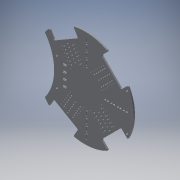
# Autodesk Inventor part: Bottom Plate
Saved by Autodesk Inventor 2016 (Build 200138000, 138)
## iProperties
Created: 2015-08-20
Part Number: Bottom Plate
Material: Generic
Document SubType Name: Modeling
Designer: TFHulbert
Density: 1 g/cm^3
Appearance: Default
Author: TFHulbert
Autodesk Inventor part; units mm, degrees
ref_plane "YZ Plane" through (0, 0, 0) normal (1, 0, 0) x (0, 1, 0)
ref_plane "XZ Plane" through (0, 0, 0) normal (0, 1, 0) x (-1, 0, 0)
ref_plane "XY Plane" through (0, 0, 0) normal (0, 0, 1) x (1, 0, 0)
sketch "Sketch1" plane through (0, 0, 0) normal (0, 1, 0) x (-1, 0, 0)
  arc A0 (31.5311, 101.5419) -> (30.2114, 104.4989) centre (29.799, 102.5419) ccw
  arc A1 (-38.945, 95.3943) -> (-39.4544, 92.1964) centre (-38.0402, 93.6107) ccw
  arc A2 (-81.8808, 49.77) -> (-85.0786, 49.2607) centre (-83.295, 48.3558) ccw
  arc A3 (30.2114, -100.9882) -> (31.5311, -98.0311) centre (29.799, -99.0311) ccw
  arc A4 (86.7133, -68.3668) -> (93.5107, -59.9572) centre (8.5603, 1.7554) ccw
  arc A5 (83.4926, -68.0311) -> (86.7133, -68.3668) centre (85.2246, -67.0311) ccw
  arc A6 (93.5107, 63.4679) -> (86.7133, 71.8775) centre (8.5603, 1.7554) ccw
  arc A7 (93.5154, 61.1235) -> (93.5107, 63.4679) centre (91.8926, 62.2924) ccw
  arc A8 (86.7133, 71.8775) -> (83.4926, 71.5419) centre (85.2246, 70.5419) ccw
  line L0 (83.4926, 71.5419) -> (75.8526, 58.309)
  arc A9 (73.1206, 57.577) -> (75.8526, 58.309) centre (74.1206, 59.309) ccw
  line L1 (31.5311, 101.5419) -> (23.8911, 88.309)
  circle A10 centre (39.3604, 23.0262) radius 1
  circle A11 centre (42.4973, 28.6048) radius 1
  circle A12 centre (45.6973, 34.1473) radius 1
  circle A13 centre (48.8973, 39.6899) radius 1
  circle A14 centre (52.0973, 45.2325) radius 1
  circle A15 centre (55.2973, 50.775) radius 1
  circle A16 centre (58.4973, 56.3176) radius 1
  circle A17 centre (11.8074, 39.1652) radius 1
  circle A18 centre (14.9442, 44.7438) radius 1
  circle A19 centre (18.1442, 50.2863) radius 1
  circle A20 centre (21.3442, 55.8289) radius 1
  circle A21 centre (24.5442, 61.3715) radius 1
  circle A22 centre (27.7442, 66.914) radius 1
  circle A23 centre (30.9442, 72.4566) radius 1
  line L2 (31.5311, -98.0311) -> (23.8911, -84.7983)
  arc A24 (24.6231, -82.0663) -> (23.8911, -84.7983) centre (25.6231, -83.7983) ccw
  line L3 (83.4926, -68.0311) -> (75.8526, -54.7983)
  arc A25 (75.8526, -54.7983) -> (73.1206, -54.0663) centre (74.1206, -55.7983) ccw
  line L4 (73.1206, -54.0663) -> (24.6231, -82.0663)
  arc A26 (93.5154, 61.1235) -> (93.5154, -57.6128) centre (175.9423, 1.7554) ccw
  arc A27 (93.5107, -59.9572) -> (93.5154, -57.6128) centre (91.8926, -58.7817) ccw
  line L5 (-39.4544, 92.1964) -> (-28.6498, 81.3919)
  arc A28 (-28.6498, 78.5635) -> (-28.6498, 81.3919) centre (-30.064, 79.9777) ccw
  line L6 (-81.8808, 49.77) -> (-71.0762, 38.9655)
  arc A29 (-71.0762, 38.9655) -> (-68.2478, 38.9655) centre (-69.662, 40.3797) ccw
  circle A30 centre (-4.0141, 37.0113) radius 1
  circle A31 centre (-8.5907, 41.4851) radius 1
  circle A32 centre (-13.1162, 46.0106) radius 1
  circle A33 centre (-17.6417, 50.5361) radius 1
  circle A34 centre (-22.1671, 55.0615) radius 1
  circle A35 centre (-26.6926, 59.587) radius 1
  circle A36 centre (-31.2181, 64.1125) radius 1
  circle A37 centre (-26.7344, 14.5742) radius 1
  circle A38 centre (-31.311, 19.048) radius 1
  circle A39 centre (-35.8365, 23.5735) radius 1
  circle A40 centre (-40.362, 28.0989) radius 1
  circle A41 centre (-44.8875, 32.6244) radius 1
  circle A42 centre (-49.413, 37.1499) radius 1
  circle A43 centre (-53.9385, 41.6754) radius 1
  circle A44 centre (69.3609, -28.2446) radius 2.5
  circle A45 centre (69.3609, 31.7554) radius 2.5
  arc A46 (93.5107, 63.4679) -> (86.7133, 71.8775) centre (8.5603, 1.7554) ccw
  arc A47 (86.7133, -68.3668) -> (93.5107, -59.9572) centre (8.5603, 1.7554) ccw
  line L7 (8.5603, 1.7554) -> (74.3609, 1.7554)
  line L8 (8.5603, 1.7554) -> (-72.0627, 1.7554)
  line L9 (8.5603, 1.7554) -> (113.5603, 1.7554) construction
  line L10 (8.5603, 1.7554) -> (113.5603, 1.7554) construction
  arc A48 (30.2114, 104.4989) -> (-38.945, 95.3943) centre (8.5603, 1.7554) ccw
  arc A49 (-85.0786, 49.2607) -> (-85.0786, -45.75) centre (8.5603, 1.7554) ccw
  arc A50 (-39.4544, -88.6857) -> (-38.945, -91.8835) centre (-38.0402, -90.0999) ccw
  arc A51 (-85.0786, -45.75) -> (-81.8808, -46.2593) centre (-83.295, -44.8451) ccw
  line L11 (-39.4544, -88.6857) -> (-28.6498, -77.8812)
  arc A52 (-28.6498, -77.8812) -> (-28.6498, -75.0527) centre (-30.064, -76.467) ccw
  line L12 (-81.8808, -46.2593) -> (-71.0762, -35.4548)
  arc A53 (-68.2478, -35.4548) -> (-71.0762, -35.4548) centre (-69.662, -36.869) ccw
  line L13 (-68.2478, -35.4548) -> (-28.6498, -75.0527)
  arc A54 (-91.2437, -30.866) -> (-85.0786, -45.75) centre (8.5603, 1.7554) ccw
  arc A55 (-38.945, -91.8835) -> (30.2114, -100.9882) centre (8.5603, 1.7554) ccw
  arc A56 (17.9755, 39.7629) -> (19.7255, 42.794) centre (18.8505, 41.2784) ccw
  circle A57 centre (18.8505, 41.2784) radius 1.75
  arc A58 (21.1505, 45.2621) -> (22.9005, 48.2932) centre (22.0255, 46.7777) ccw
  circle A59 centre (22.0255, 46.7777) radius 1.75
  arc A60 (24.3255, 50.7614) -> (26.0755, 53.7925) centre (25.2005, 52.2769) ccw
  arc A61 (27.5005, 56.2607) -> (29.2505, 59.2918) centre (28.3755, 57.7762) ccw
  circle A62 centre (25.2005, 52.2769) radius 1.75
  arc A63 (51.2182, 53.941) -> (49.4682, 50.9099) centre (50.3432, 52.4255) ccw
  circle A64 centre (39.3218, 55.0359) radius 1.65
  circle A65 centre (29.7968, 38.5381) radius 1.65
  circle A66 centre (32.9718, 44.0374) radius 1.65
  circle A67 centre (36.1468, 49.5366) radius 1.65
  circle A68 centre (50.3432, 52.4255) radius 1.75
  circle A69 centre (47.1682, 46.9262) radius 1.75
  circle A70 centre (37.6432, 30.4284) radius 1.75
  circle A71 centre (40.8182, 35.9277) radius 1.75
  circle A72 centre (43.9932, 41.4269) radius 1.75
  line L14 (72.0627, 1.7554) -> (72.0627, -9.0946)
  arc A73 (54.3932, 59.4403) -> (52.6432, 56.4092) centre (53.5182, 57.9247) ccw
  line L15 (72.0627, -10.7446) -> (72.0627, 14.2554)
  line L16 (72.0627, 1.7554) -> (72.0627, 12.6054)
  circle A74 centre (45.6718, 66.0344) radius 1.65
  circle A75 centre (42.4968, 60.5351) radius 1.65
  circle A76 centre (28.3755, 57.7762) radius 1.75
  circle A77 centre (31.5505, 63.2755) radius 1.75
  circle A78 centre (53.5182, 57.9247) radius 1.75
  circle A79 centre (34.7255, 68.7747) radius 1.75
  line L17 (72.0627, 1.7554) -> (73.5109, -0.753)
  arc A80 (23.8911, 88.309) -> (24.6231, 85.577) centre (25.6231, 87.309) ccw
  line L18 (73.1206, 57.577) -> (24.6231, 85.577)
  line L19 (24.6231, 85.577) -> (48.8718, 71.577)
  circle A81 centre (-39.4332, 49.7489) radius 1.65
  circle A82 centre (-34.9431, 45.2587) radius 1.65
  circle A83 centre (-29.569, 55.2289) radius 1.75
  circle A84 centre (-11.6085, 37.2684) radius 1.75
  circle A85 centre (-16.0987, 41.7585) radius 1.75
  circle A86 centre (-21.4727, 31.7883) radius 1.65
  circle A87 centre (-20.5888, 46.2487) radius 1.75
  circle A88 centre (-25.9628, 36.2785) radius 1.65
  circle A89 centre (-25.0789, 50.7388) radius 1.75
  circle A90 centre (-30.4529, 40.7686) radius 1.65
  circle A91 centre (-34.0592, 59.7191) radius 1.75
  circle A92 centre (-43.9233, 54.239) radius 1.65
  circle A93 centre (-26.9527, 21.9242) radius 1.75
  circle A94 centre (-31.4429, 26.4143) radius 1.75
  circle A95 centre (-35.933, 30.9045) radius 1.75
  arc A96 (-39.1857, 34.1571) -> (-41.6606, 36.632) centre (-40.4231, 35.3946) ccw
  circle A97 centre (-44.9133, 39.8847) radius 1.75
  circle A98 centre (-49.4034, 44.3748) radius 1.75
  circle A99 centre (-40.4231, 35.3946) radius 1.75
  line L20 (-68.2478, 38.9655) -> (-28.6498, 78.5635)
  line L21 (-48.4488, 58.7645) -> (-40.1466, 58.7645) construction
  line L22 (24.6231, 85.577) -> (48.8718, 71.577)
  circle A100 centre (39.3604, -19.5155) radius 1
  circle A101 centre (42.4973, -25.0941) radius 1
  circle A102 centre (45.6973, -30.6366) radius 1
  circle A103 centre (48.8973, -36.1792) radius 1
  circle A104 centre (52.0973, -41.7218) radius 1
  circle A105 centre (55.2973, -47.2643) radius 1
  circle A106 centre (58.4973, -52.8069) radius 1
  circle A107 centre (11.8074, -35.6545) radius 1
  circle A108 centre (14.9442, -41.2331) radius 1
  circle A109 centre (18.1442, -46.7756) radius 1
  circle A110 centre (21.3442, -52.3182) radius 1
  circle A111 centre (24.5442, -57.8608) radius 1
  circle A112 centre (27.7442, -63.4033) radius 1
  circle A113 centre (30.9442, -68.9459) radius 1
  circle A114 centre (-4.0141, -33.5006) radius 1
  circle A115 centre (-8.5907, -37.9744) radius 1
  circle A116 centre (-13.1162, -42.4999) radius 1
  circle A117 centre (-17.6417, -47.0254) radius 1
  circle A118 centre (-22.1671, -51.5508) radius 1
  circle A119 centre (-26.6926, -56.0763) radius 1
  circle A120 centre (-31.2181, -60.6018) radius 1
  circle A121 centre (-26.7344, -11.0635) radius 1
  circle A122 centre (-31.311, -15.5373) radius 1
  circle A123 centre (-35.8365, -20.0627) radius 1
  circle A124 centre (-40.362, -24.5882) radius 1
  circle A125 centre (-44.8875, -29.1137) radius 1
  circle A126 centre (-49.413, -33.6392) radius 1
  circle A127 centre (-53.9385, -38.1647) radius 1
  circle A128 centre (42.4968, -57.0244) radius 1.65
  circle A129 centre (39.3218, -51.5252) radius 1.65
  arc A130 (49.4682, -47.3992) -> (51.2182, -50.4303) centre (50.3432, -48.9148) ccw
  circle A131 centre (50.3432, -48.9148) radius 1.75
  circle A132 centre (37.6432, -26.9177) radius 1.75
  circle A133 centre (40.8182, -32.417) radius 1.75
  circle A134 centre (29.7968, -35.0274) radius 1.65
  circle A135 centre (43.9932, -37.9162) radius 1.75
  circle A136 centre (32.9718, -40.5267) radius 1.65
  circle A137 centre (47.1682, -43.4155) radius 1.75
  circle A138 centre (36.1468, -46.0259) radius 1.65
  circle A139 centre (53.5182, -54.414) radius 1.75
  arc A140 (52.6432, -52.8985) -> (54.3932, -55.9296) centre (53.5182, -54.414) ccw
  circle A141 centre (45.6718, -62.5237) radius 1.65
  arc A142 (19.7255, -39.2833) -> (17.9755, -36.2522) centre (18.8505, -37.7677) ccw
  circle A143 centre (18.8505, -37.7677) radius 1.75
  arc A144 (22.9005, -44.7825) -> (21.1505, -41.7514) centre (22.0255, -43.267) ccw
  circle A145 centre (22.0255, -43.267) radius 1.75
  arc A146 (26.0755, -50.2818) -> (24.3255, -47.2507) centre (25.2005, -48.7662) ccw
  circle A147 centre (25.2005, -48.7662) radius 1.75
  arc A148 (29.2505, -55.781) -> (27.5005, -52.75) centre (28.3755, -54.2655) ccw
  circle A149 centre (31.5505, -59.7648) radius 1.75
  circle A150 centre (34.7255, -65.264) radius 1.75
  circle A151 centre (28.3755, -54.2655) radius 1.75
  circle A152 centre (-49.4034, -40.8641) radius 1.75
  circle A153 centre (-44.9133, -36.374) radius 1.75
  arc A154 (-41.6606, -33.1213) -> (-39.1857, -30.6464) centre (-40.4231, -31.8839) ccw
  circle A155 centre (-40.4231, -31.8839) radius 1.75
  circle A156 centre (-35.933, -27.3938) radius 1.75
  circle A157 centre (-31.4429, -22.9036) radius 1.75
  circle A158 centre (-26.9527, -18.4135) radius 1.75
  circle A159 centre (-21.4727, -28.2776) radius 1.65
  circle A160 centre (-25.9628, -32.7678) radius 1.65
  circle A161 centre (-30.4529, -37.2579) radius 1.65
  circle A162 centre (-34.9431, -41.748) radius 1.65
  circle A163 centre (-39.4332, -46.2381) radius 1.65
  circle A164 centre (-43.9233, -50.7283) radius 1.65
  circle A165 centre (-11.6085, -33.7577) radius 1.75
  circle A166 centre (-16.0987, -38.2478) radius 1.75
  circle A167 centre (-20.5888, -42.738) radius 1.75
  circle A168 centre (-25.0789, -47.2281) radius 1.75
  circle A169 centre (-29.569, -51.7182) radius 1.75
  circle A170 centre (-34.0592, -56.2084) radius 1.75
  line L23 (-48.4488, -55.2538) -> (-40.1466, -55.2538) construction
  point P0 (-72.0627, -41.2446)
  point P1 (-77.5952, 29.9815)
  point P2 (48.8718, -68.0663)
  dimension "d183" = 10.85
  dimension "d184" = 3.5
  dimension "d185" = 3.3
  dimension "d186" = 3.3
  dimension "d187" = 3.3
  dimension "d188" = 3.3
  dimension "d189" = 3.3
  dimension "d190" = 3.3
  dimension "d191" = 3.3
  dimension "d192" = 3.3
  dimension "d193" = 3.3
  dimension "d194" = 3.3
  dimension "d195" = 3.3
  dimension "d196" = 3.3
  constraints: 171 centre point, 102 symmetric about line, 83 point on circle, 48 end point, 3 horizontal, 3 midpoint, 2 point on line, 1 coincident, 1 collinear, 76 other
  measures "d183" distance of L16.start L14.end
  measures "d184" diameter of A63
  measures "d185" diameter of A74
  measures "d186" diameter of A75
  measures "d187" diameter of A64
  measures "d188" diameter of A67
  measures "d189" diameter of A66
  measures "d190" diameter of A65
  measures "d191" diameter of A92
  measures "d192" diameter of A81
  measures "d193" diameter of A82
  measures "d194" diameter of A90
  measures "d195" diameter of A88
  measures "d196" diameter of A86
extrude "Extrusion8" add sketch "Sketch1" against normal blind 3
sketch "Sketch14" plane through (0, 0, 0) normal (0, 1, 0) x (1, 0, 0)
  arc A0 (85.0786, -49.2607) -> (85.0786, 45.75) centre (-8.5603, -1.7554) ccw projected
  line L0 (-8.5603, -1.7554) -> (81.4397, -1.7554)
  line L1 (81.4397, -1.7554) -> (81.4397, 38.2446)
  circle A1 centre (81.4397, 38.2446) radius 2.5
  circle A2 centre (81.4397, -41.7554) radius 2.5
  point P0 (0, 0)
  dimension "d203" = 90
  dimension "d204" = 40
  dimension "d205" = 5
  constraints: 4 end point, 2 centre point, 1 coincident, 1 horizontal, 1 symmetric about line, 1 vertical, 1 other
  measures "d203" distance of L0.start L0.end
  measures "d204" distance of L0.end L1.end
  measures "d205" diameter of A1
extrude "Extrusion9" cut sketch "Sketch14" against normal blind 3
sketch "Sketch15" plane through (0, 0, 0) normal (0, 1, 0) x (1, 0, 0)
  line L0 (-57.8698, 32.3928) -> (-57.8698, 32.0292)
  line L1 (-57.8698, 32.0292) -> (-57.8698, 18.4092)
  line L2 (-57.8698, 18.4092) -> (-57.8698, 4.7892)
  line L3 (-57.8698, 4.7892) -> (-57.8698, -8.8308)
  line L4 (-57.8698, -8.8308) -> (-57.8698, -22.4508)
  line L5 (-57.8698, -1.839) -> (-57.8698, -36.0708)
  line L6 (-57.8698, -36.0708) -> (-54.7847, -36.7468)
  line L7 (-54.7847, -36.7468) -> (-50.239, -34.4141)
  line L8 (-50.239, -34.4141) -> (-38.1725, -14.554)
  line L9 (-38.1725, -14.554) -> (-34.8422, -12.8451)
  line L10 (-34.8422, -12.8451) -> (-8.0341, -30.0588)
  line L11 (-8.0341, -30.0588) -> (-8.0341, -78.5822)
  line L12 (-8.0341, -78.5822) -> (-8.0341, -99.6831)
  line L13 (-8.0341, -99.6831) -> (-7.0952, -101.449)
  line L14 (-7.0952, -101.449) -> (-2.0952, -101.449)
  line L15 (-1.1562, -99.6831) -> (-2.0952, -101.449)
  line L16 (-1.1562, -78.5822) -> (-1.1562, -99.6831)
  line L17 (-1.1562, -30.0588) -> (-1.1562, -78.5822)
  line L18 (-1.1562, -30.0588) -> (21.4276, -7.475)
  line L19 (21.4276, -7.475) -> (24.147, -4.7556)
  line L20 (24.147, -4.7556) -> (89.8399, -4.7556)
  line L21 (89.8399, -4.7556) -> (91.6058, -3.8166)
  line L22 (91.6058, 0.1386) -> (91.6058, -3.8166)
  line L23 (89.8399, 1.0776) -> (91.6058, 0.1386)
  line L24 (24.147, 1.0776) -> (89.8399, 1.0776)
  line L25 (21.4276, 3.797) -> (24.147, 1.0776)
  line L26 (-1.1562, 26.3808) -> (21.4276, 3.797)
  line L27 (-1.1562, 26.3808) -> (-1.1562, 74.9042)
  line L28 (-1.1562, 74.9042) -> (-1.1562, 96.0051)
  line L29 (-1.1562, 96.0051) -> (-2.0952, 97.771)
  line L30 (-7.0952, 97.771) -> (-2.0952, 97.771)
  line L31 (-8.0341, 96.0051) -> (-7.0952, 97.771)
  line L32 (-8.0341, 74.9042) -> (-8.0341, 96.0051)
  line L33 (-8.0341, 74.9042) -> (-8.0341, 96.0051)
  line L34 (-8.0341, 26.3808) -> (-8.0341, 74.9042)
  line L35 (-8.0341, 26.3808) -> (-8.0341, 74.9042)
  line L36 (-8.0341, 26.3808) -> (-8.0341, 74.9042)
  line L37 (-8.0341, 26.3808) -> (-8.0341, 74.9042)
  line L38 (-34.8422, 9.1671) -> (-8.0341, 26.3808)
  line L39 (-38.1725, 10.876) -> (-34.8422, 9.1671)
  line L40 (-50.239, 30.7361) -> (-38.1725, 10.876)
  line L41 (-54.7847, 33.0688) -> (-50.239, 30.7361)
  line L42 (-57.8698, 32.3928) -> (-54.7847, 33.0688)
  line L43 (-57.8698, -1.839) -> (-57.8698, -36.0708)
  line L44 (-57.8698, -1.839) -> (-57.8698, -36.0708)
  line L45 (-57.8698, -1.839) -> (-57.8698, -36.0708)
  line L46 (-57.8698, -36.0708) -> (-54.7847, -36.7468)
  line L47 (-54.7847, -36.7468) -> (-50.239, -34.4141)
  line L48 (-50.239, -34.4141) -> (-38.1725, -14.554)
  line L49 (-38.1725, -14.554) -> (-34.8422, -12.8451)
  line L50 (-34.8422, -12.8451) -> (-8.0341, -30.0588)
  line L51 (-8.0341, -30.0588) -> (-8.0341, -78.5822)
  line L52 (-8.0341, -78.5822) -> (-8.0341, -99.6831)
  line L53 (-8.0341, -99.6831) -> (-7.0952, -101.449)
  line L54 (-7.0952, -101.449) -> (-2.0952, -101.449)
  line L55 (-1.1562, -99.6831) -> (-2.0952, -101.449)
  line L56 (-1.1562, -78.5822) -> (-1.1562, -99.6831)
  line L57 (-1.1562, -30.0588) -> (-1.1562, -78.5822)
  line L58 (-1.1562, -30.0588) -> (21.4276, -7.475)
  line L59 (21.4276, -7.475) -> (24.147, -4.7556)
  line L60 (24.147, -4.7556) -> (89.8399, -4.7556)
  line L61 (89.8399, -4.7556) -> (91.6058, -3.8166)
  line L62 (91.6058, 0.1386) -> (91.6058, -3.8166)
  line L63 (89.8399, 1.0776) -> (91.6058, 0.1386)
  line L64 (24.147, 1.0776) -> (89.8399, 1.0776)
  line L65 (21.4276, 3.797) -> (24.147, 1.0776)
  line L66 (-1.1562, 26.3808) -> (21.4276, 3.797)
  line L67 (-1.1562, 26.3808) -> (-1.1562, 74.9042)
  line L68 (-1.1562, 74.9042) -> (-1.1562, 96.0051)
  line L69 (-1.1562, 96.0051) -> (-2.0952, 97.771)
  line L70 (-7.0952, 97.771) -> (-2.0952, 97.771)
  line L71 (-8.0341, 96.0051) -> (-7.0952, 97.771)
  line L72 (-8.0341, 74.9042) -> (-8.0341, 96.0051)
  line L73 (-8.0341, 69.2148) -> (-8.0341, 83.4928)
  line L74 (-8.0341, 54.9368) -> (-8.0341, 69.2148)
  line L75 (-8.0341, 40.6588) -> (-8.0341, 54.9368)
  line L76 (-8.0341, 26.3808) -> (-8.0341, 40.6588)
  line L77 (-34.8422, 9.1671) -> (-8.0341, 26.3808)
  line L78 (-38.1725, 10.876) -> (-34.8422, 9.1671)
  line L79 (-50.239, 30.7361) -> (-38.1725, 10.876)
  line L80 (-54.7847, 33.0688) -> (-50.239, 30.7361)
  line L81 (-57.8698, 32.3928) -> (-54.7847, 33.0688)
  line L82 (-57.8698, 32.3928) -> (-57.8698, 32.0292)
  line L83 (-57.8698, 32.0292) -> (-57.8698, 18.4092)
  line L84 (-57.8698, -1.839) -> (-57.8698, 26.3808)
  line L85 (-57.8698, -1.839) -> (-57.8698, 26.3808)
  line L86 (-8.0341, 26.3808) -> (-8.0341, 40.6588)
  line L87 (-34.8422, 9.1671) -> (-8.0341, 26.3808)
  line L88 (-38.1725, 10.876) -> (-34.8422, 9.1671)
  line L89 (-50.239, 30.7361) -> (-38.1725, 10.876)
  line L90 (-54.7847, 33.0688) -> (-50.239, 30.7361)
  line L91 (-57.8698, 32.3928) -> (-54.7847, 33.0688)
  line L92 (-57.8698, 32.3928) -> (-57.8698, 32.0292)
  line L93 (-57.8698, 32.0292) -> (-57.8698, 18.4092)
  line L94 (-57.8698, -1.839) -> (-57.8698, 26.3808)
  line L95 (-57.8698, -1.839) -> (-57.8698, 26.3808)
  line L96 (-57.8698, -1.839) -> (-57.8698, -36.0708)
  line L97 (-57.8698, -1.839) -> (-57.8698, -36.0708)
  line L98 (-57.8698, -1.839) -> (-57.8698, -36.0708)
  line L99 (-57.8698, -36.0708) -> (-54.7847, -36.7468)
  line L100 (-54.7847, -36.7468) -> (-50.239, -34.4141)
  line L101 (-50.239, -34.4141) -> (-38.1725, -14.554)
  line L102 (-38.1725, -14.554) -> (-34.8422, -12.8451)
  line L103 (-34.8422, -12.8451) -> (-8.0341, -30.0588)
  line L104 (-8.0341, -30.0588) -> (-8.0341, -78.5822)
  line L105 (-8.0341, -78.5822) -> (-8.0341, -99.6831)
  line L106 (-8.0341, -99.6831) -> (-7.0952, -101.449)
  line L107 (-7.0952, -101.449) -> (-2.0952, -101.449)
  line L108 (-1.1562, -99.6831) -> (-2.0952, -101.449)
  line L109 (-1.1562, -78.5822) -> (-1.1562, -99.6831)
  line L110 (-1.1562, -30.0588) -> (-1.1562, -78.5822)
  line L111 (-1.1562, -30.0588) -> (21.4276, -7.475)
  line L112 (21.4276, -7.475) -> (24.147, -4.7556)
  line L113 (24.147, -4.7556) -> (89.8399, -4.7556)
  line L114 (89.8399, -4.7556) -> (91.6058, -3.8166)
  line L115 (91.6058, 0.1386) -> (91.6058, -3.8166)
  line L116 (89.8399, 1.0776) -> (91.6058, 0.1386)
  line L117 (24.147, 1.0776) -> (89.8399, 1.0776)
  line L118 (21.4276, 3.797) -> (24.147, 1.0776)
  line L119 (-1.1562, 26.3808) -> (21.4276, 3.797)
  line L120 (-1.1562, 26.3808) -> (-1.1562, 74.9042)
  line L121 (-1.1562, 74.9042) -> (-1.1562, 96.0051)
  line L122 (-1.1562, 96.0051) -> (-2.0952, 97.771)
  line L123 (-7.0952, 97.771) -> (-2.0952, 97.771)
  line L124 (-8.0341, 96.0051) -> (-7.0952, 97.771)
  line L125 (-8.0341, 74.9042) -> (-8.0341, 96.0051)
  line L126 (-8.0341, 69.2148) -> (-8.0341, 83.4928)
  line L127 (-8.0341, 54.9368) -> (-8.0341, 69.2148)
  line L128 (-8.0341, 26.3808) -> (-8.0341, 74.9042)
  line L129 (-57.8698, -1.839) -> (-57.8698, 26.3808)
  line L130 (-57.8698, -1.839) -> (-57.8698, 26.3808)
  line L131 (-57.8698, -1.839) -> (-57.8698, 26.3808)
  line L132 (-57.8698, -1.839) -> (-57.8698, -36.0708)
  line L133 (-57.8698, -1.839) -> (-57.8698, -36.0708)
  line L134 (-57.8698, -1.839) -> (-57.8698, -36.0708)
  line L135 (-57.8698, -36.0708) -> (-54.7847, -36.7468)
  line L136 (-54.7847, -36.7468) -> (-50.239, -34.4141)
  line L137 (-50.239, -34.4141) -> (-38.1725, -14.554)
  line L138 (-38.1725, -14.554) -> (-34.8422, -12.8451)
  line L139 (-34.8422, -12.8451) -> (-8.0341, -30.0588)
  line L140 (-8.0341, -30.0588) -> (-8.0341, -78.5822)
  line L141 (-8.0341, -78.5822) -> (-8.0341, -99.6831)
  line L142 (-8.0341, -99.6831) -> (-7.0952, -101.449)
  line L143 (-7.0952, -101.449) -> (-2.0952, -101.449)
  line L144 (-1.1562, -99.6831) -> (-2.0952, -101.449)
  line L145 (-1.1562, -78.5822) -> (-1.1562, -99.6831)
  line L146 (-1.1562, -30.0588) -> (-1.1562, -78.5822)
  line L147 (-1.1562, -30.0588) -> (21.4276, -7.475)
  line L148 (21.4276, -7.475) -> (24.147, -4.7556)
  line L149 (24.147, -4.7556) -> (89.8399, -4.7556)
  line L150 (89.8399, -4.7556) -> (91.6058, -3.8166)
  line L151 (91.6058, 0.1386) -> (91.6058, -3.8166)
  line L152 (89.8399, 1.0776) -> (91.6058, 0.1386)
  line L153 (24.147, 1.0776) -> (89.8399, 1.0776)
  line L154 (21.4276, 3.797) -> (24.147, 1.0776)
  line L155 (-1.1562, 26.3808) -> (21.4276, 3.797)
  line L156 (-1.1562, 26.3808) -> (-1.1562, 74.9042)
  line L157 (-1.1562, 74.9042) -> (-1.1562, 96.0051)
  line L158 (-1.1562, 96.0051) -> (-2.0952, 97.771)
  line L159 (-7.0952, 97.771) -> (-2.0952, 97.771)
  line L160 (-8.0341, 96.0051) -> (-7.0952, 97.771)
  line L161 (-8.0341, 74.9042) -> (-8.0341, 96.0051)
  line L162 (-8.0341, 69.2148) -> (-8.0341, 83.4928)
  line L163 (-8.0341, 54.9368) -> (-8.0341, 69.2148)
  line L164 (-8.0341, 40.6588) -> (-8.0341, 54.9368)
  line L165 (-8.0341, 26.3808) -> (-8.0341, 40.6588)
  line L166 (-34.8422, 9.1671) -> (-8.0341, 26.3808)
  line L167 (-38.1725, 10.876) -> (-34.8422, 9.1671)
  line L168 (-50.239, 30.7361) -> (-38.1725, 10.876)
  line L169 (-54.7847, 33.0688) -> (-50.239, 30.7361)
  line L170 (-57.8698, 32.3928) -> (-54.7847, 33.0688)
  line L171 (-57.8698, 32.3928) -> (-57.8698, 32.0292)
  line L172 (-57.8698, 26.3808) -> (-57.8698, 32.0292)
  line L173 (-57.8698, 32.0292) -> (-57.8698, 32.3928)
  line L174 (-57.8698, 32.3928) -> (-54.7847, 33.0688)
  line L175 (-54.7847, 33.0688) -> (-50.239, 30.7361)
  line L176 (-50.239, 30.7361) -> (-38.1725, 10.876)
  line L177 (-38.1725, 10.876) -> (-34.8422, 9.1671)
  line L178 (-34.8422, 9.1671) -> (-8.0341, 26.3808)
  line L179 (-8.0341, 26.3808) -> (-8.0341, 74.9042)
  line L180 (-8.0341, 74.9042) -> (-8.0341, 96.0051)
  line L181 (-8.0341, 96.0051) -> (-7.0952, 97.771)
  line L182 (-7.0952, 97.771) -> (-2.0952, 97.771)
  line L183 (-2.0952, 97.771) -> (-1.1562, 96.0051)
  line L184 (-1.1562, 96.0051) -> (-1.1562, 74.9042)
  line L185 (-1.1562, 74.9042) -> (-1.1562, 26.3808)
  line L186 (-1.1562, 26.3808) -> (21.4276, 3.797)
  line L187 (21.4276, 3.797) -> (24.147, 1.0776)
  line L188 (24.147, 1.0776) -> (89.8399, 1.0776)
  line L189 (89.8399, 1.0776) -> (91.6058, 0.1386)
  line L190 (91.6058, 0.1386) -> (91.6058, -3.8166)
  line L191 (91.6058, -3.8166) -> (89.8399, -4.7556)
  line L192 (89.8399, -4.7556) -> (24.147, -4.7556)
  line L193 (24.147, -4.7556) -> (21.4276, -7.475)
  line L194 (21.4276, -7.475) -> (-1.1562, -30.0588)
  line L195 (-57.8698, 32.0292) -> (-57.8698, 26.3808)
  line L196 (-57.8698, 26.3808) -> (-57.8698, -1.839)
  line L197 (-57.8698, -1.839) -> (-57.8698, -36.0708)
  line L198 (-57.8698, -36.0708) -> (-54.7847, -36.7468)
  line L199 (-54.7847, -36.7468) -> (-50.239, -34.4141)
  line L200 (-50.239, -34.4141) -> (-38.1725, -14.554)
  line L201 (-38.1725, -14.554) -> (-34.8422, -12.8451)
  line L202 (-34.8422, -12.8451) -> (-8.0341, -30.0588)
  line L203 (-8.0341, -30.0588) -> (-8.0341, -78.5822)
  line L204 (-8.0341, -78.5822) -> (-8.0341, -99.6831)
  line L205 (-8.0341, -99.6831) -> (-7.0952, -101.449)
  line L206 (-7.0952, -101.449) -> (-2.0952, -101.449)
  line L207 (-2.0952, -101.449) -> (-1.1562, -99.6831)
  line L208 (-1.1562, -99.6831) -> (-1.1562, -78.5822)
  line L209 (-1.1562, -78.5822) -> (-1.1562, -30.0588)
  line L210 (77.614, -1.839) -> (78.114, -1.839)
  line L211 (78.114, -1.839) -> (78.614, -1.839)
  line L212 (64.1222, -1.839) -> (64.6222, -1.839)
  line L213 (64.6222, -1.839) -> (65.1222, -1.839)
  line L214 (51.6304, -1.839) -> (51.1304, -1.839)
  line L215 (51.1304, -1.839) -> (50.6304, -1.839)
  line L216 (38.1386, -1.839) -> (37.6386, -1.839)
  line L217 (37.6386, -1.839) -> (37.1386, -1.839)
  line L218 (-57.8698, -22.4508) -> (-55.8698, -22.4508)
  line L219 (-55.8698, -22.4508) -> (-55.8698, -22.9508)
  line L220 (-55.8698, -22.4508) -> (-55.8698, -21.9508)
  line L221 (-57.8698, -8.8308) -> (-55.8698, -8.8308)
  line L222 (-55.8698, -8.8308) -> (-55.8698, -9.3308)
  line L223 (-55.8698, -8.8308) -> (-55.8698, -8.3308)
  line L224 (-57.8698, 4.7892) -> (-55.8698, 4.7892)
  line L225 (-55.8698, 4.7892) -> (-55.8698, 4.2892)
  line L226 (-55.8698, 4.7892) -> (-55.8698, 5.2892)
  line L227 (-55.8698, 18.4092) -> (-55.8698, 18.9092)
  line L228 (-55.8698, 18.4092) -> (-55.8698, 17.9092)
  line L229 (-57.8698, 18.4092) -> (-55.8698, 18.4092)
  line L230 (-6.0341, -87.1708) -> (-6.0341, -87.6708)
  line L231 (-6.0341, -44.3368) -> (-6.0341, -43.8368)
  line L232 (-8.0341, -87.1708) -> (-6.0341, -87.1708)
  line L233 (-6.0341, -87.1708) -> (-6.0341, -86.6708)
  line L234 (-6.0341, -72.8928) -> (-6.0341, -73.3928)
  line L235 (-8.0341, -72.8928) -> (-6.0341, -72.8928)
  line L236 (-8.0341, -58.6148) -> (-6.0341, -58.6148)
  line L237 (-6.0341, -44.3368) -> (-6.0341, -44.8368)
  line L238 (-8.0341, -44.3368) -> (-6.0341, -44.3368)
  line L239 (-6.0341, -58.6148) -> (-6.0341, -58.1148)
  line L240 (-6.0341, -58.6148) -> (-6.0341, -59.1148)
  line L241 (-6.0341, -72.8928) -> (-6.0341, -72.3928)
  line L242 (-8.0341, 83.4928) -> (-6.0341, 83.4928)
  line L243 (-6.0341, 83.4928) -> (-6.0341, 82.9928)
  line L244 (-6.0341, 83.4928) -> (-6.0341, 83.9928)
  line L245 (-8.0341, 69.2148) -> (-6.0341, 69.2148)
  line L246 (-6.0341, 69.2148) -> (-6.0341, 68.7148)
  line L247 (-6.0341, 69.2148) -> (-6.0341, 69.7148)
  line L248 (-8.0341, 54.9368) -> (-6.0341, 54.9368)
  line L249 (-6.0341, 54.9368) -> (-6.0341, 54.4368)
  line L250 (-6.0341, 54.9368) -> (-6.0341, 55.4368)
  line L251 (-6.0341, 40.6588) -> (-6.0341, 41.1588)
  line L252 (-6.0341, 40.6588) -> (-6.0341, 40.1588)
  line L253 (-8.0341, 40.6588) -> (-6.0341, 40.6588)
  arc A0 (-93.5154, -61.1235) -> (-93.5154, 57.6128) centre (-175.9423, -1.7554) ccw projected
  arc A1 (85.0786, -49.2607) -> (85.0786, 45.75) centre (-8.5603, -1.7554) ccw projected
  arc A2 (-30.2114, -104.4989) -> (38.945, -95.3943) centre (-8.5603, -1.7554) ccw projected
  line L254 (78.614, -1.839) -> (78.614, -0.439)
  line L255 (78.614, -0.439) -> (83.614, -0.439)
  line L256 (83.614, -0.439) -> (83.614, -3.239)
  line L257 (83.614, -3.239) -> (78.614, -3.239)
  line L258 (78.614, -3.239) -> (78.614, -1.839)
  line L259 (78.114, -1.839) -> (78.114, -1.2219)
  line L260 (77.614, -1.839) -> (77.614, -0.439)
  line L261 (77.614, -0.439) -> (72.614, -0.439)
  line L262 (72.614, -0.439) -> (72.614, -3.239)
  line L263 (72.614, -3.239) -> (77.614, -3.239)
  line L264 (77.614, -3.239) -> (77.614, -1.839)
  line L265 (65.1222, -1.839) -> (65.1222, -0.439)
  line L266 (65.1222, -0.439) -> (70.1222, -0.439)
  line L267 (70.1222, -0.439) -> (70.1222, -3.239)
  line L268 (70.1222, -3.239) -> (65.1222, -3.239)
  line L269 (65.1222, -3.239) -> (65.1222, -1.839)
  line L270 (64.1222, -1.839) -> (64.1222, -0.439)
  line L271 (59.9222, -3.239) -> (64.1222, -3.239)
  line L272 (64.1222, -0.439) -> (59.9222, -0.439)
  line L273 (59.9222, -0.439) -> (59.9222, -3.239)
  line L274 (64.1222, -3.239) -> (64.1222, -1.839)
  line L275 (51.6304, -1.839) -> (51.6304, -0.439)
  line L276 (51.6304, -0.439) -> (56.6304, -0.439)
  line L277 (56.6304, -0.439) -> (56.6304, -3.239)
  line L278 (56.6304, -3.239) -> (51.6304, -3.239)
  line L279 (51.6304, -3.239) -> (51.6304, -1.839)
  line L280 (50.6304, -1.839) -> (50.6304, -0.439)
  line L281 (46.4304, -3.239) -> (50.6304, -3.239)
  line L282 (50.6304, -0.439) -> (46.4304, -0.439)
  line L283 (46.4304, -0.439) -> (46.4304, -3.239)
  line L284 (50.6304, -3.239) -> (50.6304, -1.839)
  line L285 (38.1386, -1.839) -> (38.1386, -0.439)
  line L286 (38.1386, -0.439) -> (43.1386, -0.439)
  line L287 (43.1386, -0.439) -> (43.1386, -3.239)
  line L288 (43.1386, -3.239) -> (38.1386, -3.239)
  line L289 (38.1386, -3.239) -> (38.1386, -1.839)
  line L290 (37.1386, -1.839) -> (37.1386, -0.439)
  line L291 (32.9386, -3.239) -> (37.1386, -3.239)
  line L292 (37.1386, -0.439) -> (32.9386, -0.439)
  line L293 (32.9386, -0.439) -> (32.9386, -3.239)
  line L294 (37.1386, -3.239) -> (37.1386, -1.839)
  line L295 (-6.0341, -59.1148) -> (-6.0341, -61.4148)
  line L296 (-6.0341, -61.4148) -> (-6.0341, -63.5148)
  line L297 (-6.0341, -61.4148) -> (-6.0341, -67.9148)
  line L298 (-6.0341, -67.9148) -> (-3.8341, -67.9148)
  line L299 (-3.8341, -67.9148) -> (-3.8341, -59.1148)
  line L300 (-6.0341, -59.1148) -> (-3.8341, -59.1148)
  line L301 (-6.0341, -43.8368) -> (-5.3341, -43.8368)
  line L302 (-5.3341, -43.8368) -> (-2.7341, -43.8368)
  line L303 (-6.0341, -43.8368) -> (-6.0341, -40.4368)
  line L304 (-6.0341, -40.4368) -> (-2.7341, -40.4368)
  line L305 (-2.7341, -40.4368) -> (-2.7341, -43.8368)
  line L306 (-6.0341, -58.1148) -> (-5.3341, -58.1148)
  line L307 (-5.3341, -58.1148) -> (-2.7341, -58.1148)
  line L308 (-6.0341, -58.1148) -> (-6.0341, -54.7148)
  line L309 (-6.0341, -54.7148) -> (-2.7341, -54.7148)
  line L310 (-2.7341, -54.7148) -> (-2.7341, -58.1148)
  line L311 (-6.0341, -72.3928) -> (-5.3341, -72.3928)
  line L312 (-5.3341, -72.3928) -> (-2.7341, -72.3928)
  line L313 (-6.0341, -72.3928) -> (-6.0341, -68.9928)
  line L314 (-6.0341, -68.9928) -> (-2.7341, -68.9928)
  line L315 (-2.7341, -68.9928) -> (-2.7341, -72.3928)
  line L316 (-6.0341, -86.6708) -> (-5.3341, -86.6708)
  line L317 (-5.3341, -86.6708) -> (-2.7341, -86.6708)
  line L318 (-6.0341, -86.6708) -> (-6.0341, -83.2708)
  line L319 (-6.0341, -83.2708) -> (-2.7341, -83.2708)
  line L320 (-2.7341, -83.2708) -> (-2.7341, -86.6708)
  line L321 (-55.8698, -22.9508) -> (-55.8698, -25.1508)
  line L322 (-55.8698, -25.1508) -> (-53.7698, -25.1508)
  line L323 (-53.7698, -25.1508) -> (-47.1198, -25.1508)
  line L324 (-47.1198, -25.1508) -> (-47.1198, -22.9508)
  line L325 (-47.1198, -22.9508) -> (-55.8698, -22.9508)
  line L326 (-55.8698, -21.9508) -> (-54.8198, -21.9508)
  line L327 (-54.8198, -21.9508) -> (-48.6198, -21.9508)
  line L328 (-55.8698, -21.9508) -> (-55.8698, -20.6508)
  line L329 (-55.8698, -20.6508) -> (-48.6198, -20.6508)
  line L330 (-48.6198, -20.6508) -> (-48.6198, -21.9508)
  line L331 (-6.0341, 40.1588) -> (-6.0341, 36.7588)
  line L332 (-6.0341, 36.7588) -> (-2.9341, 36.7588)
  line L333 (-2.9341, 36.7588) -> (-2.9341, 40.1588)
  line L334 (-2.9341, 40.1588) -> (-6.0341, 40.1588)
  line L335 (-6.0341, -73.3928) -> (-3.8341, -73.3928)
  line L336 (-6.0341, -73.3928) -> (-6.0341, -75.6928)
  line L337 (-6.0341, -75.6928) -> (-6.0341, -77.7928)
  line L338 (-3.8341, -82.1928) -> (-3.8341, -73.3928)
  line L339 (-6.0341, -75.6928) -> (-6.0341, -82.1928)
  line L340 (-6.0341, -82.1928) -> (-3.8341, -82.1928)
  line L341 (-6.0341, -87.6708) -> (-3.8341, -87.6708)
  line L342 (-6.0341, -87.6708) -> (-6.0341, -89.9708)
  line L343 (-6.0341, -89.9708) -> (-6.0341, -92.0708)
  line L344 (-3.8341, -96.4708) -> (-3.8341, -87.6708)
  line L345 (-6.0341, -89.9708) -> (-6.0341, -96.4708)
  line L346 (-6.0341, -96.4708) -> (-3.8341, -96.4708)
  line L347 (-6.0341, -44.8368) -> (-3.8341, -44.8368)
  line L348 (-6.0341, -44.8368) -> (-6.0341, -47.1368)
  line L349 (-6.0341, -47.1368) -> (-6.0341, -49.2368)
  line L350 (-3.8341, -53.6368) -> (-3.8341, -44.8368)
  line L351 (-6.0341, -47.1368) -> (-6.0341, -53.6368)
  line L352 (-6.0341, -53.6368) -> (-3.8341, -53.6368)
  line L353 (-55.8698, -9.3308) -> (-55.8698, -11.5308)
  line L354 (-55.8698, -11.5308) -> (-53.7698, -11.5308)
  line L355 (-53.7698, -11.5308) -> (-47.1198, -11.5308)
  line L356 (-47.1198, -11.5308) -> (-47.1198, -9.3308)
  line L357 (-47.1198, -9.3308) -> (-55.8698, -9.3308)
  line L358 (-55.8698, -8.3308) -> (-54.8198, -8.3308)
  line L359 (-54.8198, -8.3308) -> (-48.6198, -8.3308)
  line L360 (-55.8698, -8.3308) -> (-55.8698, -7.0308)
  line L361 (-55.8698, -7.0308) -> (-48.6198, -7.0308)
  line L362 (-48.6198, -7.0308) -> (-48.6198, -8.3308)
  line L363 (-55.8698, 4.2892) -> (-55.8698, 2.0892)
  line L364 (-55.8698, 2.0892) -> (-53.7698, 2.0892)
  line L365 (-53.7698, 2.0892) -> (-47.1198, 2.0892)
  line L366 (-47.1198, 2.0892) -> (-47.1198, 4.2892)
  line L367 (-47.1198, 4.2892) -> (-55.8698, 4.2892)
  line L368 (-55.8698, 5.2892) -> (-54.8198, 5.2892)
  line L369 (-54.8198, 5.2892) -> (-48.6198, 5.2892)
  line L370 (-55.8698, 5.2892) -> (-55.8698, 6.5892)
  line L371 (-55.8698, 6.5892) -> (-48.6198, 6.5892)
  line L372 (-48.6198, 6.5892) -> (-48.6198, 5.2892)
  line L373 (-55.8698, 17.9092) -> (-55.8698, 15.7092)
  line L374 (-55.8698, 15.7092) -> (-53.7698, 15.7092)
  line L375 (-53.7698, 15.7092) -> (-47.1198, 15.7092)
  line L376 (-47.1198, 15.7092) -> (-47.1198, 17.9092)
  line L377 (-47.1198, 17.9092) -> (-55.8698, 17.9092)
  line L378 (-55.8698, 18.9092) -> (-54.8198, 18.9092)
  line L379 (-54.8198, 18.9092) -> (-48.6198, 18.9092)
  line L380 (-55.8698, 18.9092) -> (-55.8698, 20.2092)
  line L381 (-55.8698, 20.2092) -> (-48.6198, 20.2092)
  line L382 (-48.6198, 20.2092) -> (-48.6198, 18.9092)
  line L383 (-6.0341, 41.1588) -> (-6.0341, 49.8588)
  line L384 (-6.0341, 49.8588) -> (-3.8341, 49.8588)
  line L385 (-3.8341, 49.8588) -> (-3.8341, 41.1588)
  line L386 (-3.8341, 41.1588) -> (-6.0341, 41.1588)
  line L387 (-6.0341, 54.4368) -> (-6.0341, 51.0368)
  line L388 (-6.0341, 51.0368) -> (-2.9341, 51.0368)
  line L389 (-2.9341, 51.0368) -> (-2.9341, 54.4368)
  line L390 (-2.9341, 54.4368) -> (-6.0341, 54.4368)
  line L391 (-6.0341, 55.4368) -> (-6.0341, 64.1368)
  line L392 (-6.0341, 64.1368) -> (-3.8341, 64.1368)
  line L393 (-3.8341, 64.1368) -> (-3.8341, 55.4368)
  line L394 (-3.8341, 55.4368) -> (-6.0341, 55.4368)
  line L395 (-6.0341, 68.7148) -> (-6.0341, 65.3148)
  line L396 (-6.0341, 65.3148) -> (-2.9341, 65.3148)
  line L397 (-2.9341, 65.3148) -> (-2.9341, 68.7148)
  line L398 (-2.9341, 68.7148) -> (-6.0341, 68.7148)
  line L399 (-6.0341, 69.7148) -> (-6.0341, 78.4148)
  line L400 (-6.0341, 78.4148) -> (-3.8341, 78.4148)
  line L401 (-3.8341, 78.4148) -> (-3.8341, 69.7148)
  line L402 (-3.8341, 69.7148) -> (-6.0341, 69.7148)
  line L403 (-6.0341, 82.9928) -> (-6.0341, 79.5928)
  line L404 (-6.0341, 79.5928) -> (-2.9341, 79.5928)
  line L405 (-2.9341, 79.5928) -> (-2.9341, 82.9928)
  line L406 (-2.9341, 82.9928) -> (-6.0341, 82.9928)
  line L407 (-6.0341, 83.9928) -> (-6.0341, 92.6928)
  line L408 (-6.0341, 92.6928) -> (-3.8341, 92.6928)
  line L409 (-3.8341, 92.6928) -> (-3.8341, 83.9928)
  line L410 (-3.8341, 83.9928) -> (-6.0341, 83.9928)
  point P0 (0, 0)
  dimension "d220" = 2.3
  dimension "d221" = 2.1
  dimension "d222" = 6.5
  dimension "d223" = 2.2
  dimension "d232" = 0.7
  dimension "d233" = 2.6
  dimension "d234" = 3.4
  dimension "d235" = 0.7
  dimension "d236" = 2.6
  dimension "d237" = 3.4
  dimension "d239" = 2.6
  dimension "d240" = 3.4
  dimension "d241" = 0.7
  dimension "d242" = 2.6
  dimension "d243" = 3.4
  dimension "d244" = 2.2
  dimension "d249" = 1.3
  dimension "d268" = 3.4
  dimension "d269" = 3.1
  dimension "d270" = 5
  dimension "d271" = 5
  dimension "d272" = 5
  dimension "d273" = 5
  dimension "d274" = 8.8
  dimension "d275" = 2.3
  dimension "d276" = 2.1
  dimension "d277" = 6.5
  dimension "d278" = 2.2
  dimension "d279" = 8.8
  dimension "d280" = 2.3
  dimension "d281" = 2.1
  dimension "d282" = 6.5
  dimension "d283" = 2.2
  dimension "d284" = 8.8
  dimension "d285" = 2.3
  dimension "d286" = 2.1
  dimension "d287" = 6.5
  dimension "d288" = 2.2
  dimension "d289" = 8.8
  dimension "d291" = 8.75
  dimension "d292" = 7.25
  dimension "d293" = 2.2
  dimension "d294" = 1.3
  dimension "d295" = 8.75
  dimension "d296" = 7.25
  dimension "d297" = 2.2
  dimension "d298" = 1.3
  dimension "d299" = 8.75
  dimension "d300" = 7.25
  dimension "d301" = 2.2
  dimension "d302" = 1.3
  dimension "d303" = 8.75
  dimension "d304" = 7.25
  dimension "d305" = 8.7
  dimension "d306" = 2.2
  dimension "d307" = 3.4
  dimension "d308" = 3.1
  dimension "d309" = 8.7
  dimension "d310" = 2.2
  dimension "d311" = 3.4
  dimension "d312" = 3.1
  dimension "d313" = 8.7
  dimension "d314" = 2.2
  dimension "d315" = 3.4
  constraints: 822 end point, 109 point on line, 60 perpendicular, 33 vertical, 28 horizontal, 4 collinear, 4 symmetric about line
  measures "d220" distance of L300.start L295.end
  measures "d221" distance of L295.end L296.end
  measures "d222" distance of L295.end L297.end
  measures "d223" distance of L297.end L299.start
  measures "d232" distance of L231.end L301.end
  measures "d233" distance of L301.end L302.end
  measures "d234" distance of L231.end L303.end
  measures "d235" distance of L308.start L306.end
  measures "d236" distance of L306.end L310.end
  measures "d237" distance of L308.start L308.end
  measures "d239" distance of L311.end L315.end
  measures "d240" distance of L313.start L313.end
  measures "d241" distance of L318.start L316.end
  measures "d242" distance of L316.end L320.end
  measures "d243" distance of L318.start L318.end
  measures "d244" distance of L219.end L321.end
  measures "d249" distance of L220.end L328.end
  measures "d268" distance of L252.end L331.end
  measures "d269" distance of L331.end L332.end
  measures "d270" distance of L256.end L257.end
  measures "d271" distance of L267.end L268.end
  measures "d272" distance of L277.end L278.end
  measures "d273" distance of L287.end L288.end
  measures "d274" distance of L297.end L240.end
  measures "d275" distance of L335.start L337.start
  measures "d276" distance of L337.start L337.end
  measures "d277" distance of L337.start L340.start
  measures "d278" distance of L340.start L340.end
  measures "d279" distance of L340.start point (-6.034, -73.393)
  measures "d280" distance of L341.start L343.start
  measures "d281" distance of L343.start L343.end
  measures "d282" distance of L343.start L346.start
  measures "d283" distance of L346.start L346.end
  measures "d284" distance of L346.start point (-6.034, -87.671)
  measures "d285" distance of L347.start L349.start
  measures "d286" distance of L349.start L349.end
  measures "d287" distance of L349.start L352.start
  measures "d288" distance of L352.start L352.end
  measures "d289" distance of L352.start point (-6.034, -44.837)
  measures "d291" distance of L323.end L321.end
  measures "d292" distance of L329.end L328.end
  measures "d293" distance of L353.start L353.end
  measures "d294" distance of L360.start L361.start
  measures "d295" distance of L356.start L353.end
  measures "d296" distance of L362.start L361.start
  measures "d297" distance of L363.start L363.end
  measures "d298" distance of L370.start L371.start
  measures "d299" distance of L366.start L363.end
  measures "d300" distance of L372.start L371.start
  measures "d301" distance of L373.start L373.end
  measures "d302" distance of L380.start L381.start
  measures "d303" distance of L376.start L373.end
  measures "d304" distance of L382.start L381.start
  measures "d305" distance of L251.end L383.end
  measures "d306" distance of L383.end L384.end
  measures "d307" distance of L387.start L387.end
  measures "d308" distance of L387.end L389.start
  measures "d309" distance of L394.end L392.start
  measures "d310" distance of L392.start L392.end
  measures "d311" distance of L395.start L395.end
  measures "d312" distance of L395.end L397.start
  measures "d313" distance of L402.end L400.start
  measures "d314" distance of L400.start L400.end
  measures "d315" distance of L403.start L403.end
extrude "Extrusion10" cut sketch "Sketch15" against normal through all contours L380 L381 L382 L379 L378 | L377 L376 L375 L374 L373 | L370 L371 L372 L369 L368 | L367 L366 L365 L364 L363 | L360 L361 L362 L359 L358 | L357 L356 L355 L354 L353 | L328 L329 L330 L327 L326 | L325 L324 L323 L322 L321 | L303 L304 L305 L302 L301 | L347 L350 L352 L351 L349 L348 | L308 L309 L310 L307 L306 | L300 L299 L298 L297 L296 L295 | L313 L314 L315 L312 L311 | L335 L338 L340 L339 L337 L336 | L318 L319 L320 L317 L316 | L341 L344 L346 L345 L343 L342 | L407 L408 L409 L410 | L406 L405 L404 L403 | L399 L400 L401 L402 | L398 L397 L396 L395 | L391 L392 L393 L394 | L390 L389 L388 L387 | L383 L384 L385 L386 | L334 L333 L332 L331 | L254 L255 L256 L257 L258 | L264 L263 L262 L261 L260 | L265 L266 L267 L268 L269 | L274 L271 L273 L272 L270 | L284 L281 L283 L282 L280 | L275 L276 L277 L278 L279 | L294 L291 L293 L292 L290 | L285 L286 L287 L288 L289
body "Solid3"
